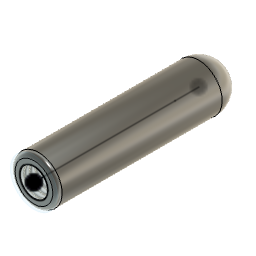
screw_v1_preparation (Autodesk Fusion 360 design; units mm, degrees)
Autodesk Fusion 360 part; units mm, degrees
sketch "Sketch1" plane through (0, 0, 0) normal (0, 1, 0) x (1, 0, 0)
  circle A0 centre (0, 0) radius 2.5
  dimension "d1" = 5
  constraint coincident A0.centre origin
  measures "d1" diameter of A0
extrude "Extrude1" add sketch "Sketch1" along normal blind 20
sketch "Sketch2" plane through (0, 0, 0) normal (0, 0, 1) x (1, 0, 0)
  line L0 (0, 0) -> (0, 15)
  line L1 (0, 15) -> (0, 17.5)
  dimension "d4" = 15
  dimension "d5" = 2.5
  constraint coincident L0.start origin
  constraint vertical L0
  constraint parallel L0 L1
  measures "d4" distance of L0.start L0.end
  measures "d5" distance of L0.end L1.end
fillet "Fillet1" radius 2.5 1 faces at (-0.8863, 20, -0.2321)
sketch "Sketch3" plane through (0, 0, 0) normal (0, -1, 0) x (1, 0, 0)
  circle A0 centre (0, 0) radius 2.5
  circle A1 centre (0, 0) radius 1.5
  dimension "d8" = 3
  constraint coincident A0.centre A1.centre
  measures "d8" diameter of A1
hole "Hole1" at (0, 0, 0) direction (0, 1, 0) diameter 2.93 depth 17.5 tip angle 180
thread "Thread1" "ISO Metric profile 3.5 M3.5x0.6 6H"
fillet "Fillet2" radius 0.5 1 edges at (-2.3308, 0, 0.904)
